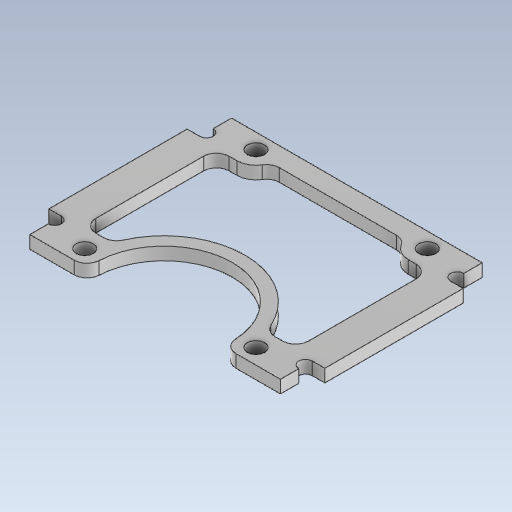
# Autodesk Inventor part: Ankle_back_frame
Saved by Autodesk Inventor 2020.4 (Build 244396000, 396)
## iProperties
Part Number: Ankle_back_frame
Material: アルミニウム 2014-T4
Document SubType Name: Modeling
Designer: Masato Kubotera
Density: 2.8 g/cm^3
Appearance: 滑らか - 淡い灰色
Description: A2017 T2
Mass: 2.81179 g
Surface Area: 16.3822 cm^2
Volume: 1.00421 cm^3
Author: Masato Kubotera
Autodesk Inventor part; units mm, degrees
ref_plane "YZ Plane" through (0, 0, 0) normal (1, 0, 0) x (0, 1, 0)
ref_plane "XZ Plane" through (0, 0, 0) normal (0, 1, 0) x (-1, 0, 0)
ref_plane "XY Plane" through (0, 0, 0) normal (0, 0, 1) x (1, 0, 0)
sketch "スケッチ1" plane through (0, 0, 0) normal (0, 0, 1) x (1, 0, 0)
  circle A0 centre (0, 0) radius 10.5 construction
  line L0 (-13.5, 28) -> (13.5, 28) construction
  line L1 (13.5, 28) -> (13.5, 1) construction
  line L2 (13.5, 1) -> (-13.5, 1) construction
  line L3 (-13.5, 1) -> (-13.5, 28) construction
  line L4 (-13.5, 28) -> (13.5, 1) construction
  line L5 (13.5, 28) -> (-13.5, 1) construction
  line L6 (-13.5, 14.5) -> (13.5, 14.5) construction
  line L7 (0, 28) -> (0, 1) construction
  circle A1 centre (-13.5, 28) radius 1.35
  circle A2 centre (-13.5, 1) radius 2.4 construction
  circle A3 centre (-13.5, 28) radius 2.4 construction
  line L8 (-19.75, 30.4) -> (19.75, 30.4)
  line L9 (-21.75, 25.4) -> (-21.75, 3.6)
  line L10 (-21.75, 25.4) -> (-19.75, 25.4)
  arc A4 (-19.75, 25.4) -> (-19.75, 27.5) centre (-19.75, 26.45) ccw
  line L11 (-19.75, 27.5) -> (-19.75, 30.4)
  line L12 (-21.75, 3.6) -> (-19.75, 3.6)
  arc A5 (-19.75, 1.5) -> (-19.75, 3.6) centre (-19.75, 2.55) ccw
  line L13 (-19.75, 1.5) -> (-19.75, -1.4)
  line L14 (-19.75, -1.4) -> (-10.6584, -1.4)
  line L15 (21.75, 25.4) -> (21.75, 3.6)
  arc A6 (19.75, 27.5) -> (19.75, 25.4) centre (19.75, 26.45) ccw
  line L16 (19.75, 27.5) -> (19.75, 30.4)
  arc A7 (19.75, 3.6) -> (19.75, 1.5) centre (19.75, 2.55) ccw
  line L17 (21.75, 3.6) -> (19.75, 3.6)
  line L18 (19.75, 1.5) -> (19.75, -1.4)
  line L19 (19.75, -1.4) -> (10.6584, -1.4)
  line L20 (21.75, 25.4) -> (19.75, 25.4)
  arc A8 (10.6584, -1.4) -> (-10.6584, -1.4) centre (0, 0) ccw
  circle A9 centre (13.5, 28) radius 1.35
  line L21 (10.5606, 27.4) -> (-10.5606, 27.4)
  arc A10 (-13.5, 25) -> (-10.5606, 27.4) centre (-13.5, 28) ccw
  line L22 (-13.5, 25) -> (-16.75, 25)
  line L23 (-16.75, 25) -> (-16.75, 4)
  arc A11 (12.1063, 4) -> (-12.1063, 4) centre (0, 0) ccw
  line L24 (-16.75, 4) -> (-12.1063, 4)
  arc A12 (10.5606, 27.4) -> (13.5, 25) centre (13.5, 28) ccw
  line L25 (13.5, 25) -> (16.75, 25)
  line L26 (16.75, 25) -> (16.75, 4)
  line L27 (16.75, 4) -> (12.1063, 4)
  line L28 (-13.5, 2.35) -> (-13.5, 2.35)
  line L29 (-13.5, -0.35) -> (-13.5, -0.35)
  arc A13 (-13.5, -0.35) -> (-13.5, 2.35) centre (-13.5, 1) ccw
  arc A14 (-13.5, 2.35) -> (-13.5, -0.35) centre (-13.5, 1) ccw
  line L30 (13.5, -0.35) -> (13.5, -0.35)
  arc A15 (13.5, 2.35) -> (13.5, -0.35) centre (13.5, 1) ccw
  arc A16 (13.5, -0.35) -> (13.5, 2.35) centre (13.5, 1) ccw
  line L31 (13.5, 2.35) -> (13.5, 2.35)
  point P0 (0, 14.5)
  dimension "d0" = 21
  dimension "d3" = 27
  dimension "d4" = 27
  dimension "d6" = 1
  dimension "d7" = 4.8
  dimension "d8" = 2
  dimension "d9" = 1.05
  dimension "d10" = 39.5
  dimension "d11" = 5
  dimension "d12" = 5
  dimension "d13" = 21.8
  dimension "d14" = 0.25
  dimension "d15" = 3
  dimension "d16" = 3
  dimension "d17" = 3
  dimension "d18" = 2
  dimension "d24" = 2.7
  dimension "d25" = 1.35
  dimension "d26" = 0
  constraints: 64 end point, 32 symmetric about line, 26 point on circle, 17 centre point, 7 tangent, 6 horizontal, 6 midpoint, 6 point on line, 5 coincident, 4 parallel, 4 perpendicular, 2 vertical, 1 concentric, 8 other
  measures "d0" diameter of A0
  measures "d3" distance of L1.end L2.end
  measures "d4" distance of L0.end L1.end
  measures "d6" distance of point (0, 0) L7.end
  measures "d7" diameter of A2
  measures "d8" distance of L9.start L10.end
  measures "d9" radius of A4
  measures "d10" distance of L8.start L8.end
  measures "d11" vertical distance of L9.start L8.start
  measures "d12" vertical distance of L9.end L13.end
  measures "d13" distance of L9.start L9.end
  measures "d14" radial gap between concentric circles of A0 A8
  measures "d15" distance between parallel lines of L21 L8
  measures "d16" radius of A10
  measures "d17" distance between parallel lines of L11 L23
  measures "d18" radial gap between concentric circles of A11 A8
  measures "d24" diameter of A1
  measures "d25" radius of A14
  measures "d26" distance of A13.centre L2.end
extrude "押し出し1" add sketch "スケッチ1" along normal blind 2
fillet "フィレット1" radius 2 2 edges at (-10.6584, -1.4, 1) (10.6584, -1.4, 1)
fillet "フィレット2" radius 2 8 edges at (-16.75, 4, 1) (-16.75, 25, 1) (-10.5606, 27.4, 1) (10.5606, 27.4, 1) (16.75, 25, 1) (16.75, 4, 1) (12.1063, 4, 1) (-12.1063, 4, 1)
equation "\"d25\" = 0.5 * d24"
